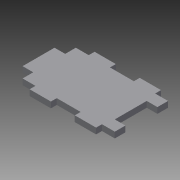
# Autodesk Inventor part: lado
Saved by Autodesk Inventor 2015 (Build 190159000, 159)
## iProperties
Created: 2017-11-28
Part Number: lado
Material: Generic
Document SubType Name: Modeling
Designer: Max
Density: 1 g/cm^3
Appearance: Default
Author: Max
Autodesk Inventor part; units mm, degrees
ref_plane "YZ Plane" through (0, 0, 0) normal (1, 0, 0) x (0, 1, 0)
ref_plane "XZ Plane" through (0, 0, 0) normal (0, 1, 0) x (-1, 0, 0)
ref_plane "XY Plane" through (0, 0, 0) normal (0, 0, 1) x (1, 0, 0)
sketch "Sketch1" plane through (0, 0, 0) normal (0, 0, 1) x (1, 0, 0)
  line L0 (-12.089, 0) -> (-12.089, -5.5)
  line L1 (-12.089, -5.5) -> (-32.089, -5.5)
  line L2 (-32.089, -5.5) -> (-32.089, 0)
  line L3 (-54.514, 0) -> (-54.514, -5.5)
  line L4 (-54.514, -5.5) -> (-74.514, -5.5)
  line L5 (-74.514, -5.5) -> (-74.514, 0)
  line L6 (-74.514, 0) -> (-86.603, 0)
  line L7 (0, 0) -> (-12.089, 0)
  line L8 (-32.089, 0) -> (-54.514, 0)
  line L9 (-12.089, 50) -> (-12.089, 55.5)
  line L10 (-12.089, 55.5) -> (-32.089, 55.5)
  line L11 (-32.089, 55.5) -> (-32.089, 50)
  line L12 (-54.514, 50) -> (-54.514, 55.5)
  line L13 (-54.514, 55.5) -> (-74.514, 55.5)
  line L14 (-74.514, 55.5) -> (-74.514, 50)
  line L15 (-32.089, 50) -> (-54.514, 50)
  line L16 (-86.603, 50) -> (-74.514, 50)
  line L17 (-12.089, 50) -> (0, 50)
  line L18 (-86.603, 10) -> (-96.603, 10)
  line L19 (-96.603, 10) -> (-96.603, 40)
  line L20 (-96.603, 40) -> (-86.603, 40)
  line L21 (-86.603, 0) -> (-86.603, 10)
  line L22 (-86.603, 40) -> (-86.603, 50)
  line L23 (0, 10) -> (-10, 10)
  line L24 (-10, 10) -> (-10, 40)
  line L25 (-10, 40) -> (0, 40)
  line L26 (0, 50) -> (0, 40)
  line L27 (0, 10) -> (0, 0)
  dimension "d2" = 5.5
  dimension "d3" = 20
  dimension "d4" = 5.5
  dimension "d5" = 20
  dimension "d6" = 90
  dimension "d8" = 30
  dimension "d11" = 10
  dimension "d12" = 10
  dimension "d13" = 30
  dimension "d14" = 10
  dimension "d15" = 90
  constraints: 56 end point, 19 perpendicular, 13 parallel, 4 horizontal, 1 vertical
  measures "d2" distance of L0.start L0.end
  measures "d3" distance of L0.end L1.end
  measures "d4" distance of L3.start L3.end
  measures "d5" distance of L3.end L4.end
  measures "d6" angle of L3 L4
  measures "d8" distance of L18.end L19.end
  measures "d11" distance between parallel lines of L22 L19
  measures "d12" distance of L23.start L23.end
  measures "d13" distance of L23.end L24.end
  measures "d14" distance of L24.end L25.end
  measures "d15" angle of L24 L25
extrude "Extrusion1" add sketch "Sketch1" along normal blind 5.5
body "Solid1"
